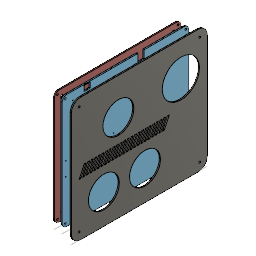
PC2 v62 (Autodesk Fusion 360 design; units mm, degrees)
Autodesk Fusion 360 part; units mm, degrees
sketch "Sketch1" plane through (0, 0, 0) normal (1, 0, 0) x (0, 0, -1)
  line L0 (15, 0) -> (395, 0)
  line L1 (410, -15) -> (410, -355)
  line L2 (395, -370) -> (15, -370)
  line L3 (0, -355) -> (0, -15)
  line L4 (0, -20) -> (245, -20)
  line L5 (245, -20) -> (245, -265)
  line L6 (245, -265) -> (0, -265)
  line L7 (0, -265) -> (0, -20)
  line L8 (71, -20) -> (91, -20)
  line L9 (91, -20) -> (91, -3)
  line L10 (91, -3) -> (71, -3)
  line L11 (71, -3) -> (71, -20)
  line L12 (245, -146) -> (261, -146)
  line L13 (261, -146) -> (261, -93)
  line L14 (261, -93) -> (245, -93)
  line L15 (245, -93) -> (245, -146)
  line L16 (245, -20) -> (265, -20)
  line L17 (265, -20) -> (265, 0.4081)
  line L18 (265, 0.4081) -> (245, 0.4081)
  line L19 (245, 0.4081) -> (245, -20)
  line L20 (220, -265) -> (170, -265)
  line L21 (170, -265) -> (170, -280)
  line L22 (170, -280) -> (220, -280)
  line L23 (220, -280) -> (220, -265)
  circle A0 centre (90, -288) radius 50
  circle A1 centre (137, -103) radius 50
  circle A2 centre (10, -360) radius 3
  circle A3 centre (400, -360) radius 3
  circle A4 centre (10, -10) radius 3
  circle A5 centre (400, -10) radius 3
  arc A6 (0, -355) -> (15, -370) centre (15, -355) ccw
  arc A7 (395, -370) -> (410, -355) centre (395, -355) ccw
  arc A8 (15, 0) -> (0, -15) centre (15, -15) ccw
  arc A9 (410, -15) -> (395, 0) centre (395, -15) ccw
  arc A10 (425, -15) -> (395, 15) centre (395, -15) ccw
  line L24 (15, 15) -> (395, 15)
  arc A11 (15, 15) -> (-15, -15) centre (15, -15) ccw
  line L25 (-15, -355) -> (-15, -15)
  arc A12 (-15, -355) -> (15, -385) centre (15, -355) ccw
  line L26 (395, -385) -> (15, -385)
  arc A13 (395, -385) -> (425, -355) centre (395, -355) ccw
  line L27 (425, -15) -> (425, -355)
  circle A14 centre (339, -95) radius 60
  circle A15 centre (90, -288) radius 57.5
  circle A16 centre (90, -288) radius 68
  circle A17 centre (137, -103) radius 57.5
  circle A18 centre (137, -103) radius 68
  line L28 (303, -178) -> (10, -178)
  line L29 (10, -178) -> (10, -213)
  line L30 (10, -213) -> (303, -213)
  line L31 (303, -213) -> (303, -178)
  line L32 (10, -213) -> (26.3208, -178)
  line L33 (10, -213) -> (56.3399, -213) construction
  line L34 (15.8529, -213) -> (32.1737, -178)
  line L35 (21.7059, -213) -> (38.0267, -178)
  line L36 (27.5588, -213) -> (43.8796, -178)
  line L37 (33.4118, -213) -> (49.7325, -178)
  line L38 (39.2647, -213) -> (55.5855, -178)
  line L39 (45.1176, -213) -> (61.4384, -178)
  line L40 (50.9706, -213) -> (67.2914, -178)
  line L41 (56.8235, -213) -> (73.1443, -178)
  line L42 (62.6765, -213) -> (78.9972, -178)
  line L43 (68.5294, -213) -> (84.8502, -178)
  line L44 (74.3824, -213) -> (90.7031, -178)
  line L45 (80.2353, -213) -> (96.5561, -178)
  line L46 (86.0882, -213) -> (102.409, -178)
  line L47 (91.9412, -213) -> (108.2619, -178)
  line L48 (97.7941, -213) -> (114.1149, -178)
  line L49 (103.6471, -213) -> (119.9678, -178)
  line L50 (109.5, -213) -> (125.8208, -178)
  line L51 (115.3529, -213) -> (131.6737, -178)
  line L52 (121.2059, -213) -> (137.5267, -178)
  line L53 (127.0588, -213) -> (143.3796, -178)
  line L54 (132.9118, -213) -> (149.2325, -178)
  line L55 (138.7647, -213) -> (155.0855, -178)
  line L56 (144.6176, -213) -> (160.9384, -178)
  line L57 (150.4706, -213) -> (166.7914, -178)
  line L58 (156.3235, -213) -> (172.6443, -178)
  line L59 (162.1765, -213) -> (178.4972, -178)
  line L60 (168.0294, -213) -> (184.3502, -178)
  line L61 (173.8824, -213) -> (190.2031, -178)
  line L62 (179.7353, -213) -> (196.0561, -178)
  line L63 (185.5882, -213) -> (201.909, -178)
  line L64 (191.4412, -213) -> (207.7619, -178)
  line L65 (197.2941, -213) -> (213.6149, -178)
  line L66 (203.1471, -213) -> (219.4678, -178)
  line L67 (209, -213) -> (225.3208, -178)
  circle A19 centre (238.5, -26.5) radius 1.5
  circle A20 centre (166.5, -26.5) radius 1.5
  circle A21 centre (34.5, -26.5) radius 1.5
  circle A22 centre (238.5, -184) radius 1.5
  circle A23 centre (166.5, -184) radius 1.5
  circle A24 centre (11.5, -184) radius 1.5
  circle A25 centre (11.5, -229) radius 1.5
  circle A26 centre (166.5, -250) radius 1.5
  line L68 (383, -19) -> (383, -20.4174)
  line L69 (387, -20.4174) -> (387, -19)
  arc A27 (387, -19) -> (383, -19) centre (385, -19) ccw
  arc A28 (383, -20.4174) -> (387, -20.4174) centre (385, -25) ccw
  arc A29 (383, -340.4174) -> (387, -340.4174) centre (385, -345) ccw
  line L70 (387, -340.4174) -> (387, -339)
  line L71 (383, -339) -> (383, -340.4174)
  arc A30 (387, -339) -> (383, -339) centre (385, -339) ccw
  arc A31 (27, -339) -> (23, -339) centre (25, -339) ccw
  line L72 (23, -339) -> (23, -340.4174)
  line L73 (27, -340.4174) -> (27, -339)
  arc A32 (23, -340.4174) -> (27, -340.4174) centre (25, -345) ccw
  arc A33 (27, -19) -> (23, -19) centre (25, -19) ccw
  arc A34 (23, -20.4174) -> (27, -20.4174) centre (25, -25) ccw
  line L74 (23, -19) -> (23, -20.4174)
  line L75 (27, -20.4174) -> (27, -19)
  line L76 (265, -20) -> (245, -20)
  line L77 (245, -20) -> (245, -26.0663)
  line L78 (245, -26.0663) -> (265, -26.0663)
  line L79 (265, -26.0663) -> (265, -20)
  circle A35 centre (223, -288) radius 50
  line L80 (214.853, -213) -> (231.1738, -178)
  line L81 (209.0001, -213) -> (225.3208, -178)
  line L82 (220.706, -213) -> (237.0268, -178)
  line L83 (214.8531, -213) -> (231.1738, -178)
  line L84 (226.559, -213) -> (242.8798, -178)
  line L85 (220.7061, -213) -> (237.0268, -178)
  line L86 (232.412, -213) -> (248.7328, -178)
  line L87 (226.5591, -213) -> (242.8798, -178)
  line L88 (238.265, -213) -> (254.5858, -178)
  line L89 (232.4121, -213) -> (248.7328, -178)
  line L90 (244.118, -213) -> (260.4388, -178)
  line L91 (238.2651, -213) -> (254.5858, -178)
  line L92 (249.971, -213) -> (266.2918, -178)
  line L93 (244.1181, -213) -> (260.4388, -178)
  line L94 (255.824, -213) -> (272.1448, -178)
  line L95 (249.9711, -213) -> (266.2918, -178)
  line L96 (261.677, -213) -> (277.9978, -178)
  line L97 (255.8241, -213) -> (272.1448, -178)
  line L98 (267.53, -213) -> (283.8508, -178)
  line L99 (261.6771, -213) -> (277.9978, -178)
  line L100 (273.383, -213) -> (289.7038, -178)
  line L101 (267.5301, -213) -> (283.8508, -178)
  line L102 (279.236, -213) -> (295.5568, -178)
  line L103 (273.3831, -213) -> (289.7038, -178)
  line L104 (285.089, -213) -> (301.4098, -178)
  line L105 (279.2361, -213) -> (295.5568, -178)
  line L106 (245, -241.8305) -> (265, -241.8305)
  line L107 (265, -241.8305) -> (265, -213.8305)
  line L108 (265, -213.8305) -> (245, -213.8305)
  line L109 (245, -213.8305) -> (245, -241.8305)
  point P0 (410, 0)
  point P1 (0, -370)
  dimension "d2" = 410
  dimension "d3" = 370
  dimension "d4" = 245
  dimension "d5" = 245
  dimension "d6" = 20
  dimension "d7" = 71
  dimension "d8" = 20
  dimension "d9" = 17
  dimension "d10" = 53
  dimension "d11" = 16
  dimension "d12" = 73
  dimension "d14" = 20
  dimension "d15" = 75
  dimension "d16" = 50
  dimension "d17" = 15
  dimension "d18" = 90
  dimension "d19" = 268
  dimension "d20" = 83
  dimension "d21" = 137
  dimension "d22" = 100
  dimension "d23" = 100
  dimension "d24" = 6
  dimension "d25" = 10
  dimension "d26" = 10
  dimension "d27" = 6
  dimension "d28" = 10
  dimension "d29" = 10
  dimension "d30" = 6
  dimension "d31" = 10
  dimension "d32" = 10
  dimension "d33" = 6
  dimension "d34" = 10
  dimension "d35" = 10
  dimension "d36" = 15
  dimension "d37" = 15
  dimension "d38" = 15
  dimension "d39" = 15
  dimension "d40" = -15
  dimension "d57" = 339
  dimension "d58" = 75
  dimension "d59" = 120
  dimension "d60" = 115
  dimension "d61" = 136
  dimension "d62" = 115
  dimension "d63" = 136
  dimension "d68" = 65
  dimension "d71" = 199
  dimension "d72" = 0
  dimension "d73" = 3
  dimension "d74" = 6.5
  dimension "d75" = 6.5
  dimension "d76" = 3
  dimension "d77" = 72
  dimension "d78" = 3
  dimension "d79" = 132
  dimension "d80" = 3
  dimension "d81" = 157.5
  dimension "d82" = 3
  dimension "d83" = 72
  dimension "d84" = 3
  dimension "d85" = 155
  dimension "d86" = 3
  dimension "d87" = 45
  dimension "d88" = 3
  dimension "d89" = 66
  dimension "d90" = 10
  dimension "d91" = 25
  dimension "d92" = 25
  dimension "d93" = 4
  dimension "d94" = 4
  dimension "d95" = 6
  dimension "d96" = 10
  dimension "d97" = 4
  dimension "d98" = 4
  dimension "d99" = 6
  dimension "d100" = 25
  dimension "d101" = 10
  dimension "d102" = 4
  dimension "d103" = 4
  dimension "d104" = 6
  dimension "d105" = 25
  dimension "d106" = 10
  dimension "d107" = 4
  dimension "d108" = 4
  dimension "d109" = 6
  dimension "d110" = 25
  dimension "d113" = 133
  dimension "d114" = 75
  dimension "d115" = 75
  dimension "d116" = 80
  dimension "d117" = 80
  dimension "d120" = 5.853
  dimension "d121" = 0
  dimension "d122" = 28
  dimension "d123" = 20
  constraint horizontal L0
  constraint vertical L1
  constraint horizontal L2
  constraint vertical L3
  constraint horizontal L4
  constraint vertical L5
  constraint horizontal L6
  constraint vertical L7
  constraint coincident L3 L4.start
  constraint horizontal L8
  constraint vertical L9
  constraint horizontal L10
  constraint vertical L11
  constraint coincident L4 L8.start
  constraint horizontal L12
  constraint vertical L13
  constraint horizontal L14
  constraint vertical L15
  constraint coincident L5 L12.start
  constraint horizontal L16
  constraint vertical L17
  constraint horizontal L18
  constraint vertical L19
  constraint horizontal L20
  constraint vertical L21
  constraint horizontal L22
  constraint vertical L23
  constraint coincident L6 L20.start
  constraint equal A0 A1
  constraint tangent L2 A6
  constraint tangent L3 A6
  constraint tangent L2 A7
  constraint tangent L1 A7
  constraint tangent L3 A8
  constraint tangent L0 A8
  constraint tangent L1 A9
  constraint tangent L0 A9
  constraint horizontal L28
  constraint vertical L29
  constraint horizontal L30
  constraint vertical L31
  constraint horizontal L33
  constraint coincident L28 L32.end
  constraint vertical A28.centre A27.centre
  constraint vertical L68
  constraint vertical L69
  constraint vertical A29.centre A30.centre
  constraint vertical L71
  constraint vertical L70
  constraint vertical A32.centre A31.centre
  constraint vertical L72
  constraint vertical L73
  constraint vertical A33.centre A34.centre
  constraint vertical L74
  constraint vertical L75
  constraint coincident L5 L77.end
  constraint equal A0 A35
  constraint horizontal A0.centre A35.centre
  constraint coincident A0.centre A15.centre
  constraint horizontal L106
  constraint vertical L107
  constraint horizontal L108
  constraint vertical L109
  constraint coincident L5 L106.start
  constraint coincident A1.centre A17.centre
  measures "d2" distance of origin P0
  measures "d3" distance of origin P1
  measures "d4" distance of L4.start L4.end
  measures "d5" distance of L4.start L6.end
  measures "d6" distance of L0 L4
  measures "d7" distance of L3 L11
  measures "d8" distance of L9.end L10.end
  measures "d9" distance of L8 L10
  measures "d10" distance of L12.start L14.end
  measures "d11" distance of L12.start L12.end
  measures "d12" distance of L4 L14
  measures "d14" distance of L4.end L16.end
  measures "d15" distance of L5 L21
  measures "d16" distance of L21.end L22.end
  measures "d17" distance of L20.start L22.end
  measures "d18" distance of L3 A0.centre
  measures "d19" distance of L4 A0.centre
  measures "d20" distance of L4 A1.centre
  measures "d21" distance of L7 A1.centre
  measures "d22" diameter of A1
  measures "d23" diameter of A0
  measures "d24" diameter of A2
  measures "d25" distance of L3 A2.centre
  measures "d26" distance of L2 A2.centre
  measures "d27" diameter of A3
  measures "d28" distance of L1 A3.centre
  measures "d29" distance of L2 A3.centre
  measures "d30" diameter of A4
  measures "d31" distance of L3 A4.centre
  measures "d32" distance of L0 A4.centre
  measures "d33" diameter of A5
  measures "d34" distance of L0 A5.centre
  measures "d35" distance of L1 A5.centre
  measures "d36" radius of A6
  measures "d37" radius of A7
  measures "d38" radius of A8
  measures "d39" radius of A9
  measures "d40" distance of A9
  measures "d57" distance of L7 A14.centre
  measures "d58" distance of L4 A14.centre
  measures "d59" diameter of A14
  measures "d60" diameter of A15
  measures "d61" diameter of A16
  measures "d62" diameter of A17
  measures "d63" diameter of A18
  measures "d68" angle of L32 L33
  measures "d73" diameter of A19
  measures "d74" distance of L4 A19.centre
  measures "d75" distance of L5 A19.centre
  measures "d76" diameter of A20
  measures "d77" distance of A19.centre A20.centre
  measures "d78" diameter of A21
  measures "d79" distance of A20.centre A21.centre
  measures "d80" diameter of A22
  measures "d81" distance of A19.centre A22.centre
  measures "d82" diameter of A23
  measures "d83" distance of A22.centre A23.centre
  measures "d84" diameter of A24
  measures "d85" distance of A23.centre A24.centre
  measures "d86" diameter of A25
  measures "d87" distance of A24.centre A25.centre
  measures "d88" diameter of A26
  measures "d89" distance of A23.centre A26.centre
  measures "d90" diameter of A28
  measures "d91" distance of L0 A28.centre
  measures "d92" distance of L1 A28.centre
  measures "d93" diameter of A27
  measures "d94" distance of L69.end L68.start
  measures "d95" distance of A28.centre A27.centre
  measures "d96" diameter of A29
  measures "d97" diameter of A30
  measures "d98" distance of L71.start L70.end
  measures "d99" distance of A29.centre A30.centre
  measures "d100" distance of L2 A29.centre
  measures "d101" diameter of A32
  measures "d102" diameter of A31
  measures "d103" distance of A31.end A31.start
  measures "d104" distance of A32.centre A31.centre
  measures "d105" distance of L3 A32.centre
  measures "d106" diameter of A34
  measures "d107" diameter of A33
  measures "d108" distance of A33.start A33.end
  measures "d109" distance of A33.centre A34.centre
  measures "d110" distance of L0 A34.centre
  measures "d113" distance of A0.centre A35.centre
  measures "d114" distance of A0.centre L30
  measures "d115" distance of A1.centre L28
  measures "d116" distance of A0.centre L29
  measures "d117" distance of L31 A35.centre
  measures "d122" distance of L106.start L108.end
  measures "d123" distance of L106.start L106.end
extrude "Extrude1" add sketch "Sketch1" along normal blind 4 contours L0 L3 L4 L9 L10 L11 L19 A8 A33 L74 L75 | L0 L16 L17 L19 L76 | L0 L1 L2 L3 L5 L6 L12 L13 L14 L17 L21 L22 A6 A7 A9 A16 L28 L30 L31 L78 L79 A35 L106 L107 L108 | L3 L4 L5 L6 L7 L8 L15 L20 A16 L28 L29 L30 A34 L74 L75 L77 A35 L109 | L5 L16 L76 L77 L78 L79 | L4 L8 L9 L10 L11 | L5 L12 L13 L14 L15 | L6 A15 A16 | L6 A15 A16 | L6 A0 A15 | L6 A0 A15 | L5 L28 L86 L89 | L5 L28 L30 A22 L84 L86 L87 L89 | L6 A0 | L6 A0 | L6 L20 L21 L22 A35 | L5 L28 L86 L88 L89 L91 | L5 L30 L86 L88 L89 L91 | L28 L30 A22 L82 L84 L85 L87 | L5 L6 L20 A35 | L6 L20 L22 L23 A35 | L5 L28 L88 L90 L91 L93 | L5 L30 L88 L90 L91 L93 | L28 L30 L80 L82 L83 L85 | A22 L84 L87 | A22 L84 L87 | L5 L6 L22 L23 A35 | L5 L28 L30 L90 L92 L93 L95 | L5 L30 L90 L93 | L28 L30 L67 L80 L81 L83 | L5 L106 L107 L108 L109 | L28 L30 L92 L94 L95 L97 | L28 L30 L66 L67 L81 | L28 L30 L94 L96 L97 L99 | L28 L30 L65 L66 | L28 L30 L96 L98 L99 L101 | L28 L30 L64 L65 | L28 L30 L98 L100 L101 L103 | L28 L30 L63 L64 | L28 L30 L100 L102 L103 L105 | L28 L30 L62 L63 | L28 L30 L102 L104 L105 | L28 L30 L61 L62 | L28 L30 L31 L104 | L28 L30 L60 L61 | L28 L30 L59 L60 | L28 L30 L58 L59 | L28 L30 L57 L58 | L28 L30 L56 L57 | L28 L30 L55 L56 | L28 L30 L54 L55 | L28 L30 L53 L54 | L28 L30 L52 L53 | L28 L30 L51 L52 | L28 L30 L50 L51 | L28 L30 L49 L50 | L28 L30 L48 L49 | L28 L30 L47 L48 | L28 L30 L46 L47 | L28 L30 L45 L46 | L28 L30 L44 L45 | L28 L30 L43 L44 | L28 L30 L42 L43 | L28 L30 L41 L42 | L28 L30 L40 L41 | L28 L30 L39 L40 | L28 L30 L38 L39 | L28 L30 L37 L38 | L28 L30 L36 L37 | L28 L30 L35 L36 | L28 L30 L34 L35 | L28 L30 L32 L34 | A24 | L28 L29 L32 | A1 | A14 | A17 | A18 | A19 | A20 | A21 | A23 | A25 | A26 makes body 1
extrude "Extrude2" add sketch "Sketch1" along normal blind 4 separate body contours L0 L3 L4 L9 L10 L11 L19 A8 A33 L74 L75 | L0 L1 L2 L3 L5 L6 L12 L13 L14 L17 L21 L22 A6 A7 A9 A16 L28 L30 L31 L78 L79 A35 L106 L107 L108 | L3 L4 L5 L6 L7 L8 L15 L20 A16 L28 L29 L30 A34 L74 L75 L77 A35 L109 | L4 A33 L74 L75 | L4 A34 L74 L75 | L6 A15 A16 | L6 A15 A16 | L6 A0 A15 | L6 A0 A15 | L5 L28 L86 L89 | L5 L28 L30 A22 L84 L86 L87 L89 | L6 A0 | L6 A0 | L5 L28 L86 L88 L89 L91 | L5 L30 L86 L88 L89 L91 | L28 L30 A22 L82 L84 L85 L87 | L5 L6 L20 A35 | L5 L28 L88 L90 L91 L93 | L5 L30 L88 L90 L91 L93 | L28 L30 L80 L82 L83 L85 | L5 L6 L22 L23 A35 | L5 L28 L30 L90 L92 L93 L95 | L5 L30 L90 L93 | L28 L30 L67 L80 L81 L83 | L28 L30 L92 L94 L95 L97 | L28 L30 L66 L67 L81 | L28 L30 L94 L96 L97 L99 | L28 L30 L65 L66 | L28 L30 L96 L98 L99 L101 | L28 L30 L64 L65 | L28 L30 L98 L100 L101 L103 | L28 L30 L63 L64 | L28 L30 L100 L102 L103 L105 | L28 L30 L62 L63 | L28 L30 L102 L104 L105 | L28 L30 L61 L62 | L28 L30 L31 L104 | L28 L30 L60 L61 | L28 L30 L59 L60 | L28 L30 L58 L59 | L28 L30 L57 L58 | L28 L30 L56 L57 | L28 L30 L55 L56 | L28 L30 L54 L55 | L28 L30 L53 L54 | L28 L30 L52 L53 | L28 L30 L51 L52 | L28 L30 L50 L51 | L28 L30 L49 L50 | L28 L30 L48 L49 | L28 L30 L47 L48 | L28 L30 L46 L47 | L28 L30 L45 L46 | L28 L30 L44 L45 | L28 L30 L43 L44 | L28 L30 L42 L43 | L28 L30 L41 L42 | L28 L30 L40 L41 | L28 L30 L39 L40 | L28 L30 L38 L39 | L28 L30 L37 L38 | L28 L30 L36 L37 | L28 L30 L35 L36 | L28 L30 L34 L35 | L28 L30 L32 L34 | L28 L29 L32 | A1 | A14 | A17 | A18 | L68 L69 A27 A28 | A29 L70 L71 A30 | A31 L72 L73 A32 makes body 2
extrude "Extrude3" add sketch "Sketch1" along normal blind 4 separate body contours L0 L3 L4 L9 L10 L11 L19 A8 A33 L74 L75 | L0 L17 L18 L19 | L0 L16 L17 L19 L76 | L0 L1 L2 L3 L5 L6 L12 L13 L14 L17 L21 L22 A6 A7 A9 A16 L28 L30 L31 L78 L79 A35 L106 L107 L108 | L3 L4 L5 L6 L7 L8 L15 L20 A16 L28 L29 L30 A34 L74 L75 L77 A35 L109 | L5 L16 L76 L77 L78 L79 | L4 L8 L9 L10 L11 | L4 A33 L74 L75 | L4 A34 L74 L75 | L5 L12 L13 L14 L15 | L6 A15 A16 | L6 A15 A16 | L6 A0 A15 | L6 A0 A15 | L5 L28 L86 L89 | L5 L28 L30 A22 L84 L86 L87 L89 | L6 L20 L21 L22 A35 | L5 L28 L88 L90 L91 L93 | L5 L30 L88 L90 L91 L93 | L28 L30 L80 L82 L83 L85 | A22 L84 L87 | L5 L30 L90 L93 | L5 L106 L107 L108 L109 | L28 L30 L92 L94 L95 L97 | L28 L30 L66 L67 L81 | L28 L30 L96 L98 L99 L101 | L28 L30 L64 L65 | L28 L30 L100 L102 L103 L105 | L28 L30 L62 L63 | L28 L30 L31 L104 | L28 L30 L60 L61 | L28 L30 L58 L59 | L28 L30 L56 L57 | L28 L30 L54 L55 | L28 L30 L52 L53 | L28 L30 L50 L51 | L28 L30 L48 L49 | L28 L30 L46 L47 | L28 L30 L44 L45 | L28 L30 L42 L43 | L28 L30 L40 L41 | L28 L30 L38 L39 | L28 L30 L36 L37 | L28 L30 L34 L35 | A24 | L28 L29 L32 | A10 L24 A11 L25 A12 L26 A13 L27 | A17 | A18 | A19 | A20 | A21 | A25 | A26 | L68 L69 A27 A28 | A29 L70 L71 A30 | A31 L72 L73 A32 picked at (239.8458, -184.5455) makes body 3
move_body "Move1" bodies 3 to x (1, 0, 0) y (0, 1, 0) z (0, 0, 1) at (70, 0, 0)
move_body "Move2" bodies 2 to x (1, 0, 0) y (0, 1, 0) z (0, 0, 1) at (25, 0, 0)
extrude "Extrude4" cut sketch "Sketch1" along normal blind 71 contours L6 A15 A16 | L6 A15 A16 | A18 bodies 3
